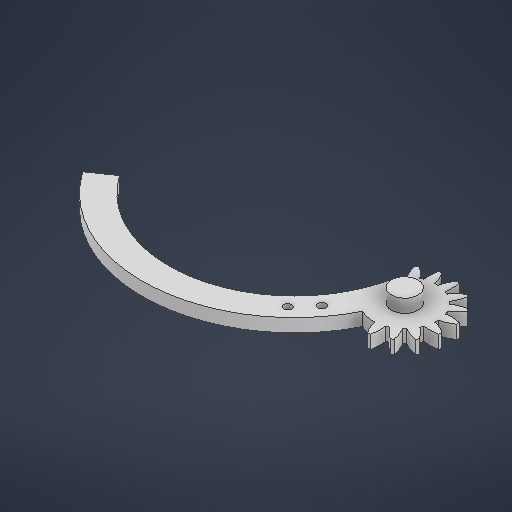
# Autodesk Inventor part: Left_Top_Gripper
Saved by Autodesk Inventor 2026.1 (Build 301233020, 233B)
## iProperties
Created: 2025-10-25
Part Number: Left_Top_Gripper
Material: Generic
Document SubType Name: Modeling
Designer: Garfieldcmix
Density: 1 g/cm^3
Appearance: Default
Author: Garfieldcmix
Autodesk Inventor part; units mm, degrees
ref_plane "YZ Plane" through (0, 0, 0) normal (1, 0, 0) x (0, 1, 0)
ref_plane "XZ Plane" through (0, 0, 0) normal (0, 1, 0) x (-1, 0, 0)
ref_plane "XY Plane" through (0, 0, 0) normal (0, 0, 1) x (1, 0, 0)
derived "Right_Top_Gripper.ipt"
sketch "Sketch14" plane through (0, 0, 0) normal (0, 1, 0) x (-1, 0, 0)
  arc A0 (-40.2823, -25.1712) -> (38.9097, -27.2449) centre (0, 0) ccw projected
  line L0 (38.9097, -27.2449) -> (47.1012, -32.9806) projected
  arc A1 (-48.7628, -30.4704) -> (47.1012, -32.9806) centre (0, 0) ccw projected
  arc A2 (-44.6354, -16.246) -> (-40.2823, -25.1712) centre (0, 0) ccw
  arc A3 (-54.0323, -19.6662) -> (-48.7628, -30.4704) centre (0, 0) ccw
  line L1 (-44.6354, -16.246) -> (-54.0323, -19.6662)
  line L2 (0, -70.9188) -> (0, 14.3646) construction
  dimension "d21" = 70
  constraints: 4 point on circle, 2 centre point, 2 coincident, 2 end point, 1 line through centre
  measures "d21" angle of L1 L2
extrude "Extrusion6" add sketch "Sketch14" along normal blind 5
sketch "Sketch5" plane through (0, 0, 0) normal (0, 1, 0) x (-1, 0, 0)
  arc A0 (-46.8208, -8.0042) -> (-44.6354, -16.246) centre (-56.5705, -15) ccw projected
  line L0 (70.3114, 0) -> (-92.1596, 0) construction
  arc A1 (-46.8208, -8.0042) -> (-44.6354, -16.246) centre (0, 0) ccw projected
  circle A2 centre (-56.5705, -15) radius 3 projected
  arc A3 (-44.6354, -16.246) -> (38.9097, -27.2449) centre (0, 0) ccw construction
extrude "Extrusion3" add sketch "Sketch5" along normal up to surface (5 mm away)
sketch "Sketch15" plane through (0, 5, 0) normal (0, 1, 0) x (1, 0, 0)
  circle A0 centre (41.9284, 31.5953) radius 1.5 projected
  circle A1 centre (35.8049, 38.3961) radius 1.5 projected
  point P0 (0, 0)
extrude "Extrusion7" cut sketch "Sketch15" against normal up to surface (5 mm away)
sketch "Sketch16" plane through (0, 0, 0) normal (0, -1, 0) x (1, 0, 0)
  arc A0 (58.3205, -3.1283) -> (57.0955, 2.1217) centre (44.3294, -3.625) ccw construction
  line L0 (56.0455, 2.1217) -> (57.0955, 2.1217) construction
  arc A1 (56.0455, 2.1217) -> (54.8205, -3.1283) centre (68.8117, -3.625) ccw construction
  line L1 (54.8205, -3.1283) -> (58.3205, -3.1283) construction
  line L2 (56.5705, -15) -> (56.5705, -3) construction
  line L3 (58.3205, -3.1283) -> (57.0955, 2.1217) construction
  line L4 (54.8205, -3.1283) -> (56.0455, 2.1217) construction
  arc A2 (51.3777, -25.8182) -> (46.8208, -8.0042) centre (56.5705, -15) ccw construction
  line L5 (56.5705, -15) -> (54.2295, -3.2306) construction
  line L6 (55.9709, -3.015) -> (52.5381, -3.6978)
  line L7 (55.9709, -3.015) -> (53.7452, 1.8951) construction
  line L8 (52.5381, -3.6978) -> (52.7153, 1.6903) construction
  line L9 (53.7452, 1.8951) -> (52.7153, 1.6903)
  arc A3 (55.9709, -3.015) -> (53.7452, 1.8951) centre (42.3454, -6.2317) ccw
  arc A4 (52.7153, 1.6903) -> (52.5381, -3.6978) centre (66.3574, -1.4554) ccw
  point P0 (0, 0)
  point P1 (52.7153, 1.6903)
  dimension "d26" = 11.25
  constraints: 10 end point, 6 point on circle, 4 equal length, 2 centre point, 2 equal radius, 1 perpendicular, 1 point on line, 1 symmetric about line
  measures "d26" angle of L5 L2
extrude "Extrusion8" add sketch "Sketch16" against normal up to surface (5 mm away)
pattern_circular "Circular Pattern1" count 2 over 22.5 about axis through (56.5705, 0, -15) along (0, -1, 0) of "Extrusion8"
pattern_circular "Circular Pattern2" count 9 over 180 about axis through (56.5705, 0, -15) along (0, 1, 0) of "Extrusion8"
mirror "Mirror1" about plane through (0, 0, 0) normal (0, 0, 1) remove original yes
sketch "Sketch17" plane through (0, 5, 0) normal (0, 1, 0) x (0.9973656, 0, -0.0725387)
  circle A0 centre (55.3334, -19.064) radius 3 construction
  circle A1 centre (55.3334, -19.064) radius 5
  point P0 (0, 0)
  dimension "d29" = 10
  constraints: 1 centre point, 1 coincident
  measures "d29" diameter of A1
extrude "Extrusion9" add sketch "Sketch17" along normal blind 5
sketch "Sketch1" plane through (0, 0, 0) normal (0, 1, 0) x (-1, 0, 0)
  arc A0 (-40.2823, -25.1712) -> (38.9097, -27.2449) centre (0, 0) ccw projected
  line L0 (-40.2823, -25.1712) -> (-48.7628, -30.4704) projected
  line L1 (38.9097, -27.2449) -> (47.1012, -32.9806) projected
  arc A1 (-48.7628, -30.4704) -> (47.1012, -32.9806) centre (0, 0) ccw projected
  line L2 (0, -70.4825) -> (0, 11.7471) construction
sketch "Sketch3" plane through (0, 17, 0) normal (0, 1, 0) x (1, 0, 0)
  circle A0 centre (41.9284, 31.5953) radius 1.5 projected
  arc A1 (40.2823, 25.1712) -> (22.2999, 41.94) centre (0, 0) ccw construction
  arc A2 (48.7628, 30.4704) -> (26.9946, 50.7695) centre (0, 0) ccw construction
  line L0 (40.2823, 25.1712) -> (48.7628, 30.4704) construction
  line L1 (26.9946, 50.7695) -> (22.2999, 41.94) construction
  line L2 (37.9352, 28.5862) -> (45.9215, 34.6044) construction
  line L3 (32.3949, 34.7393) -> (39.2149, 42.0528) construction
  circle A3 centre (35.8049, 38.3961) radius 1.5 projected
sketch "Sketch6" plane through (0, 0, 0) normal (0, 1, 0) x (-1, 0, 0)
  arc A0 (-46.8208, -8.0042) -> (-51.3777, -25.8182) centre (-56.5705, -15) ccw construction
  line L0 (-56.5705, -15) -> (-56.5705, -3) construction
  line L1 (-54.8205, -3.1283) -> (-58.3205, -3.1283) projected
  line L2 (-58.3205, -3.1283) -> (-57.0955, 2.1217) construction
  line L3 (-54.8205, -3.1283) -> (-56.0455, 2.1217) construction
  line L4 (-56.0455, 2.1217) -> (-57.0955, 2.1217) projected
  arc A1 (-54.8205, -3.1283) -> (-56.0455, 2.1217) centre (-68.8117, -3.625) ccw projected
  arc A2 (-57.0955, 2.1217) -> (-58.3205, -3.1283) centre (-44.3294, -3.625) ccw projected
  point P0 (0, 0)
body "Solid3"
body "Solid2"
